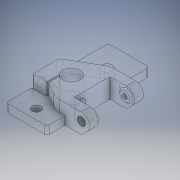
# Autodesk Inventor part: XY Idler Mount 1.0
Saved by Autodesk Inventor 2016 (Build 200138000, 138)
## iProperties
Created: 2017-01-26
Part Number: XY Idler Mount 1.0
Material: PET Plastic
Document SubType Name: Modeling
Designer: Scott
Density: 1.541 g/cm^3
Appearance: Gunmetal
Author: Scott
Autodesk Inventor part; units mm, degrees
ref_plane "YZ Plane" through (0, 0, 0) normal (1, 0, 0) x (0, 1, 0)
ref_plane "XZ Plane" through (0, 0, 0) normal (0, 1, 0) x (-1, 0, 0)
ref_plane "XY Plane" through (0, 0, 0) normal (0, 0, 1) x (1, 0, 0)
sketch "Sketch1" plane through (0, 0, 0) normal (0, 0, 1) x (1, 0, 0)
  circle A0 centre (0, 0) radius 5.2
  line L0 (-12.5, 35) -> (12.5, 35)
  line L1 (12.5, 35) -> (12.5, -27.5)
  line L2 (12.5, -27.5) -> (-12.5, -27.5)
  line L3 (-12.5, -27.5) -> (-12.5, 35)
  circle A1 centre (0, 21.5) radius 3.2
  line L4 (0, 0) -> (0, 46.1814) construction
  line L5 (0, 0) -> (0, -50.1978) construction
  circle A2 centre (0, -21.5) radius 2.7
  dimension "d0" = 10.4
  dimension "d1" = 35
  dimension "d2" = 27.5
  dimension "d3" = 12.5
  dimension "d4" = 12.5
  dimension "d5" = 13.5
  dimension "d6" = 6.4
  dimension "d7" = 5.4
  dimension "d8" = 21.5
  constraints: 12 end point, 3 centre point, 2 parallel, 2 perpendicular, 2 point on line, 1 coincident, 1 horizontal, 1 vertical
  measures "d0" diameter of A0
  measures "d1" distance from line of L0 L4.start
  measures "d2" distance from line of L2 L4.start
  measures "d3" distance from line of L1 L4.start
  measures "d4" distance from line of L3 point (0, 0)
  measures "d5" distance from line of A1.centre L0
  measures "d6" diameter of A1
  measures "d7" diameter of A2
  measures "d8" distance of point (0, 0) A2.centre
extrude "Extrusion1" add sketch "Sketch1" along normal blind 5
sketch "Sketch2" plane through (0, 0, 0) normal (0, 0, -1) x (-1, 0, 0)
  line L0 (0, 0) -> (-52.1343, 0) construction
  circle A0 centre (0, 0) radius 5.2 projected
  line L1 (12.5, -27.5) -> (12.5, 35) projected
  line L2 (-12.5, 35) -> (-12.5, -27.5) projected
  line L3 (12.5, 35) -> (12.5, -27.5) projected
  line L4 (12.5, 5) -> (-7.4186, 16.5)
  line L5 (-7.4186, 16.5) -> (-28, 16.5)
  line L6 (-28, 16.5) -> (-28, 11)
  line L7 (-28, 11) -> (-12.5, 11)
  line L8 (3, -11) -> (-6.5263, -16.5)
  line L9 (-6.5263, -16.5) -> (-28, -16.5)
  line L10 (-28, -16.5) -> (-28, -11)
  line L11 (-28, -11) -> (-12.5, -11)
  line L12 (-12.5, 11) -> (-12.5, -11)
  circle A1 centre (0, 0) radius 5.2
  line L13 (12.5, 5) -> (12.5, -5)
  line L14 (12.5, -11) -> (3, -11)
  point P0 (12.5, -7)
  dimension "d11" = 28
  dimension "d12" = 11
  dimension "d13" = 11
  dimension "d14" = 5.5
  dimension "d15" = 5.5
  dimension "d16" = 5
  dimension "d18" = 30
  dimension "d19" = 30
  dimension "d56" = 11
  dimension "d57" = 9.5
  constraints: 24 end point, 8 point on line, 4 perpendicular, 2 horizontal, 1 centre point, 1 coincident, 1 collinear, 1 concentric, 1 parallel
  measures "d11" distance from line of L0.start L6
  measures "d12" vertical distance of L0.start L6.end
  measures "d13" distance from line of L0.start L11
  measures "d14" distance of L5.end L6.end
  measures "d15" distance of L9.end L10.end
  measures "d16" vertical distance of L4.start L0.start
  measures "d18" angle of L4 L0
  measures "d19" angle of L0 L8
  measures "d56" distance from line of L14 L0.start
  measures "d57" distance of L14.start L8.start
extrude "Extrusion2" add sketch "Sketch2" against normal blind 12
fillet "Fillet1" radius 10 2 edges at (7.4186, 16.5, 8.5) (6.5263, -16.5, 8.5)
fillet "Fillet2" radius 2.5 1 edges at (-12.5, 5, 8.5)
sketch "Sketch3" plane through (12.5, -16.5, 0) normal (0, -1, 0) x (1, 0, 0)
  line L0 (15.5, 0) -> (0, 0) projected
  line L1 (15.5, 0) -> (15.5, 12) projected
  line L2 (-12.5, -21.7134) -> (-12.5, 18.9904) projected
  line L3 (10, 7) -> (10, -15.8986) construction
  line L4 (-3.2942, 12) -> (15.5, 12) projected
  line L5 (0, 12) -> (15.5, 12) projected
  line L6 (15.5, 12) -> (15.5, 0)
  line L7 (10, 0) -> (15.5, 0)
  arc A0 (13.4993, 3.4286) -> (10, 12) centre (10, 7) ccw
  line L8 (15.5, 12) -> (-3.2942, 12) projected
  line L9 (10, 12) -> (15.5, 12)
  line L10 (10, 0) -> (13.4993, 3.4286)
  circle A1 centre (10, 7) radius 1.5
  point P0 (-12.5, 0)
  dimension "d24" = 22.5
  dimension "d25" = 7
  dimension "d27" = 3
  constraints: 10 end point, 3 coincident, 3 point on line, 3 tangent, 2 centre point, 2 collinear, 2 point on circle, 1 perpendicular, 1 vertical
  measures "d24" distance from line of L3.start L2
  measures "d25" distance from line of L0 L3.start
  measures "d27" diameter of A1
extrude "Extrusion3" cut sketch "Sketch3" against normal through all contours L0 L10 A0 L4 L1
sketch "Sketch4" plane through (12.5, 11, 0) normal (0, -1, 0) x (1, 0, 0)
  circle A0 centre (10, 7) radius 4
  point P0 (-12.5, 0)
  point P1 (10, 7)
  dimension "d30" = 8
  constraints: 1 centre point, 1 coincident
  measures "d30" diameter of A0
extrude "Extrusion4" add sketch "Sketch4" along normal blind 1 draft -45
mirror "Mirror1" about plane through (0, 0, 0) normal (0, 1, 0) of "Extrusion4"
sketch "Sketch5" plane through (12.5, 16.5, 5) normal (0, 1, 0) x (1, 0, 0)
  point P0 (-12.5, 5)
  point P1 (10, -2)
hole "Hole1" at (22.5, 16.5, 7) direction (0, -1, 0) diameter 3 end through all counterbore diameter 6.2 counterbore depth 1.5
sketch "Sketch6" plane through (12.5, -16.5, 0) normal (0, -1, 0) x (1, 0, 0)
  point P0 (-12.5, 0)
  point P1 (10, 7)
hole "Hole2" at (22.5, -16.5, 7) direction (0, 1, 0) diameter 4.7 depth 5 counterbore diameter 5 counterbore depth 0.5
fillet "Fillet3" radius 1.5 4 edges at (12.5, 35, 2.5) (-12.5, 35, 2.5) (-12.5, -27.5, 2.5) (12.5, -27.5, 2.5)
sketch "Sketch8" plane through (0, 0, 12) normal (0, 0, 1) x (1, 0, 0)
  line L0 (-3, -11) -> (4.2058, -15.1603) projected
  circle A0 centre (0, 0) radius 5.2 projected
  line L1 (-12.5, -11) -> (-3, -11) projected
  line L2 (-3, -11) -> (-3, -4.2474)
  line L3 (-4, -3.3226) -> (-4, -11)
  line L4 (-12.5, -12) -> (-3, -12)
  line L5 (-3, -11) -> (-3, -12)
  line L6 (-12.5, -11) -> (-12.5, -12)
  line L7 (-12.5, -26) -> (-12.5, 33.5) projected
  line L8 (-12.5, -11) -> (-4, -11)
  dimension "d58" = 1
  dimension "d59" = 1
  constraints: 12 end point, 3 vertical, 2 collinear, 2 point on circle, 1 horizontal, 1 point on line
  measures "d58" distance between parallel lines of L2 L3
  measures "d59" distance between parallel lines of L4 L1
extrude "Extrusion5" cut sketch "Sketch8" against normal through all contours A0 L2 L1 L3 | L1 L5 L4 L6
sketch "Sketch9" plane through (12.5, -11, 0) normal (1, 0, 0) x (0, 0, -1)
  line L0 (-12, 0) -> (0, 0) projected
  line L1 (0, 22) -> (0, 0) projected
  line L2 (0, 22) -> (-12, 22) projected
  line L3 (-12, 0) -> (-12, 22) projected
  line L4 (-6, 0) -> (-6, 11.5392) construction
  point P0 (0, 11)
  point P1 (-6, 4)
  dimension "d62" = 4
  constraints: 2 end point, 1 midpoint, 1 point on line, 1 vertical
  measures "d62" distance from line of point (-6, 4) L0
hole "Hole4" at (12.5, -7, 6) direction (-1, 0, 0) diameter 3.5 end through all counterbore diameter 6.5 counterbore depth 3
hole "Hole5" at (-12.5, -7, 6) direction (1, 0, 0) diameter 4.7 depth 5 counterbore diameter 5 counterbore depth 1
fillet "Fillet5" radius 0.5 10 edges at (-12.5, -11, 6) (-3, -11, 8.5) (-4, -11, 6) (-12.5, -12, 2.5) (-4, -3.3226, 6) (-3, -4.2474, 6) (12.5, -11, 6) (12.5, 11, 6) (12.5, 16.5, 2.5) (12.5, -16.5, 2.5)
fillet "Fillet6" radius 1.5 1 edges at (-3, -12, 2.5)
equation "\"d4\" = d3"
equation "\"d13\" = d12"
equation "\"d15\" = d14"
equation "\"d19\" = d18"
body "Solid1"
